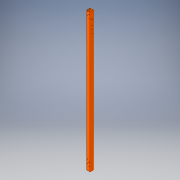
# Autodesk Inventor part: ElvFixedBeam
Saved by Autodesk Inventor 2019 (Build 230136000, 136)
## iProperties
Created: 2019-01-09
Part Number: ElvFixedBeam
Material: Aluminum 6061
Document SubType Name: Modeling
Designer: james
Density: 2.7 g/cm^3
Appearance: Default(2)
Mass: 404.32 g
Surface Area: 1890.01 cm^2
Volume: 149.748 cm^3
Author: james
Autodesk Inventor part; units mm, degrees
ref_plane "YZ Plane" through (0, 0, 0) normal (1, 0, 0) x (0, 1, 0)
ref_plane "XZ Plane" through (0, 0, 0) normal (0, 1, 0) x (-1, 0, 0)
ref_plane "XY Plane" through (0, 0, 0) normal (0, 0, 1) x (1, 0, 0)
sketch "Sketch1" plane through (0, 0, 0) normal (0, 1, 0) x (-1, 0, 0)
  line L0 (17.0295, 14.999) -> (-8.3705, 14.999)
  line L1 (-8.3705, 14.999) -> (-8.3705, -10.401)
  line L2 (-8.3705, -10.401) -> (17.0295, -10.401)
  line L3 (17.0295, -10.401) -> (17.0295, 14.999)
  line L4 (15.442, -8.8135) -> (-6.783, -8.8135)
  line L5 (-6.783, -8.8135) -> (-6.783, 13.4115)
  line L6 (-6.783, 13.4115) -> (15.442, 13.4115)
  line L7 (15.442, 13.4115) -> (15.442, -8.8135)
  point P0 (0, 0)
  dimension "d0" = 25.4
  dimension "d1" = 25.4
  dimension "d4" = 1.5875
  dimension "d5" = 1.5875
  dimension "d6" = 1.5875
  dimension "d7" = 1.5875
  constraints: 16 end point, 4 parallel, 2 horizontal, 2 perpendicular
  measures "d0" distance of L0.end L1.end
  measures "d1" distance of L0.start L0.end
  measures "d4" distance between parallel lines of L0 L6
  measures "d5" distance between parallel lines of L2 L4
  measures "d6" distance between parallel lines of L3 L7
  measures "d7" distance between parallel lines of L1 L5
extrude "Extrusion2" add sketch "Sketch1" along normal blind 990.6
sketch "Sketch4" plane through (8.3705, 0, 14.999) normal (1, 0, 0) x (0, 0, -1)
  line L0 (25.4, 0) -> (25.4, 990.6) projected
  line L1 (0, 990.6) -> (25.4, 990.6) projected
  point P0 (14.999, 0)
  point P1 (12.7, 939.8)
  dimension "d28" = 12.7
  dimension "d29" = 50.8
  measures "d28" distance from line of L0 point (12.7, 939.8)
  measures "d29" distance from line of L1 point (12.7, 939.8)
hole "Hole3" at (8.3705, 939.8, 2.299) direction (-1, 0, 0) diameter 9.5758 depth 25.4 tip angle 118
sketch "Sketch5" plane through (8.3705, 0, 14.999) normal (1, 0, 0) x (0, 0, -1)
  line L0 (0, 0) -> (0, 990.6) projected
  line L1 (0, 990.6) -> (25.4, 990.6) projected
  point P0 (14.999, 0)
  point P1 (12.7, 901.7)
  point P2 (12.7, 876.3)
  point P3 (12.7, 850.9)
  dimension "d37" = 25.4
  dimension "d38" = 25.4
  dimension "d39" = 12.7
  dimension "d40" = 12.7
  dimension "d41" = 12.7
  dimension "d42" = 88.9
  measures "d37" distance of point (12.7, 876.3) point (12.7, 901.7)
  measures "d38" distance of point (12.7, 850.9) point (12.7, 876.3)
  measures "d39" distance from line of point (12.7, 901.7) L0
  measures "d40" distance from line of L0 point (12.7, 876.3)
  measures "d41" distance from line of L0 point (12.7, 850.9)
  measures "d42" distance from line of point (12.7, 901.7) L1
hole "Hole4" at (8.3705, 901.7, 2.299) at (8.3705, 876.3, 2.299) at (8.3705, 850.9, 2.299) direction (-1, 0, 0) diameter 4.826 depth 25.4 tip angle 118
sketch "Sketch6" plane through (-17.0295, 0, 14.999) normal (0, 0, 1) x (1, 0, 0)
  line L0 (0, 0) -> (0, 990.6) projected
  line L1 (0, 990.6) -> (25.4, 990.6) projected
  line L2 (25.4, 0) -> (25.4, 990.6) projected
  point P0 (17.0295, 0)
  point P1 (6.35, 984.25)
  point P2 (19.05, 971.55)
  point P3 (6.35, 958.85)
  point P4 (19.05, 946.15)
  dimension "d50" = 6.35
  dimension "d51" = 6.35
  dimension "d52" = 6.35
  dimension "d53" = 25.4
  dimension "d54" = 6.35
  dimension "d55" = 19.05
  dimension "d56" = 6.35
  dimension "d57" = 25.4
  measures "d50" distance from line of L0 point (6.35, 984.25)
  measures "d51" distance from line of L1 point (6.35, 984.25)
  measures "d52" distance from line of L0 point (6.35, 958.85)
  measures "d53" distance of point (6.35, 958.85) point (6.35, 984.25)
  measures "d54" distance from line of L2 point (19.05, 971.55)
  measures "d55" distance from line of L1 point (19.05, 971.55)
  measures "d56" distance from line of L2 point (19.05, 946.15)
  measures "d57" distance of point (19.05, 946.15) point (19.05, 971.55)
hole "Hole5" at (-10.6795, 984.25, 14.999) at (2.0205, 971.55, 14.999) at (-10.6795, 958.85, 14.999) at (2.0205, 946.15, 14.999) direction (0, 0, -1) diameter 4.7625 depth 25.4 tip angle 118
sketch "Sketch7" plane through (-17.0295, 0, 14.999) normal (0, 0, 1) x (1, 0, 0)
  line L0 (25.4, 0) -> (25.4, 990.6) projected
  line L1 (0, 0) -> (25.4, 0) projected
  line L2 (0, 0) -> (0, 990.6) projected
  point P0 (17.0295, 0)
  point P1 (19.05, 31.75)
  point P2 (19.05, 57.15)
  point P3 (6.35, 44.45)
  point P4 (6.35, 69.85)
  dimension "d65" = 6.35
  dimension "d66" = 31.75
  dimension "d67" = 6.35
  dimension "d68" = 25.4
  dimension "d69" = 6.35
  dimension "d70" = 6.35
  dimension "d71" = 25.4
  dimension "d72" = 44.45
  measures "d65" distance from line of L0 point (19.05, 31.75)
  measures "d66" distance from line of L1 point (19.05, 31.75)
  measures "d67" distance from line of L0 point (19.05, 57.15)
  measures "d68" distance of point (19.05, 31.75) point (19.05, 57.15)
  measures "d69" distance from line of L2 point (6.35, 44.45)
  measures "d70" distance from line of L2 point (6.35, 69.85)
  measures "d71" distance of point (6.35, 44.45) point (6.35, 69.85)
  measures "d72" distance from line of L1 point (6.35, 44.45)
hole "Hole6" at (2.0205, 31.75, 14.999) at (2.0205, 57.15, 14.999) at (-10.6795, 44.45, 14.999) at (-10.6795, 69.85, 14.999) direction (0, 0, -1) diameter 4.7625 depth 25.4 tip angle 118
equation "\"d0\" = ElvBeamWidth"
equation "\"d1\" = ElvBeamWidth"
equation "\"d4\" = ElvWallWidth"
equation "\"d5\" = ElvWallWidth"
equation "\"d6\" = ElvWallWidth"
equation "\"d7\" = ElvWallWidth"
equation "\"d8\" = ElvFrontBeamLength"
equation "\"d29\" = ElvHoleFromFixed"
equation "\"ElvMiddleBeamLength\" = 990.6"
equation "\"ElvWallWidth\" = 1.5875"
equation "\"ElvFrontBeamLength\" = 990.6"
equation "\"ElvEndEffectLength\" = 431.8"
equation "\"ElvCrossBeamLength\" = 304.8"
equation "\"ElvBeamWidth\" = 25.4"
equation "\"ElvFrontBeamLength_1\" = 1066.8"
equation "\"ElvFixedBeamLength\" = 990.6"
equation "\"ElvDelHeight\" = 101.6"
equation "\"ElvDelDepth\" = 6.35"
equation "\"ElvDelFrontTabLength\" = 6.35"
equation "\"ElvDelWidth\" = 18.542"
equation "\"ElvTopBeamLength\" = 457.2"
equation "\"ElvHoleFromBottom\" = 38.1"
equation "\"ElvHoleFromFront\" = 25.4"
equation "\"ElvHoleFromMid\" = 38.1"
equation "\"ElvHoleFromFixed\" = 50.8"
equation "\"ElvRivetPlateLength\" = 76.2"
equation "\"ElvDelMiddleTabLength\" = 6.35"
body "Solid2"
